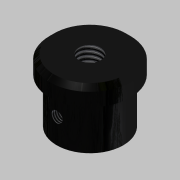
# Autodesk Inventor part: BackPair1PistonBottomCap
Saved by Autodesk Inventor 2015 SP1 (Build 190203100, 203)
## iProperties
Created: 2014-09-27
Part Number: BackPair1PistonBottomCap
Material: Generic
Document SubType Name: Modeling
Designer: Inventor
Mass: 3.17839 g
Surface Area: 17.4372 cm^2
Volume: 3.17839 cm^3
Density: 1 g/cm^3
Appearance: Glossy - Black
Author: Inventor
Autodesk Inventor part; units mm, degrees
ref_plane "YZ Plane" through (0, 0, 0) normal (1, 0, 0) x (0, 1, 0)
ref_plane "XY Plane" through (0, 0, 0) normal (0, 0, 1) x (1, 0, 0)
sketch "Mount" plane through (0, 0, 0) normal (0, 0, 1) x (1, 0, 0)
  circle A0 centre (0, 0) radius 7.45
  dimension "d0" = 14.9
  constraints: 1 centre point, 1 coincident
  measures "d0" diameter of A0
extrude "MountFeature" add sketch "Mount" along normal blind 10
sketch "Base" plane through (0, 0, 10) normal (0, 0, 1) x (1, 0, 0)
  circle A0 centre (0, 0) radius 7.45 construction
  circle A1 centre (0, 0) radius 9
  dimension "d3" = 18
  constraints: 1 centre point, 1 coincident
  measures "d3" diameter of A1
extrude "BaseFeature" add sketch "Base" along normal blind 4
sketch "RodEndHole" plane through (0, 0, 14) normal (0, 0, 1) x (1, 0, 0)
  circle A0 centre (0, 0) radius 9 projected
hole "RodEndHoleFeature" at (0, 0, 14) direction (0, 0, -1) diameter 4.917 end through all thread size "M6x1" class "6H" standard "ISO Metric profile"
chamfer "BaseChamferFeature" distance 1 angle 45 1 edges at (-9, 0, 14)
ref_plane "MidSidePlane" through (0, 12, 0) normal (0, 1, 0) x (-1, 0, 0)
sketch "MountHole" plane through (0, 12, 0) normal (0, 1, 0) x (-1, 0, 0)
  line L0 (-9, 10) -> (9, 10) construction
  line L1 (7.45, 0) -> (7.45, 10) construction
  line L2 (7.45, 10) -> (-7.45, 10) construction
  line L3 (-7.45, 0) -> (7.45, 0) construction
  point P0 (0, 5.5)
  dimension "d18" = 4.5
  dimension "d26" = 18
  dimension "d27" = 9
  measures "d18" distance from line of L0 point (0, 5.5)
  measures "d26" distance of L0.start L0.end
  measures "d27" horizontal distance of L0.end point (0, 5.5)
hole "MountHoleFeature" at (0, 12, 5.5) direction (0, -1, 0) diameter 2.459 end through all thread size "M3x0.5" class "6H" standard "ISO Metric profile"
equation "\"d27\" = 0.5 * d26"
body "Solid1"
